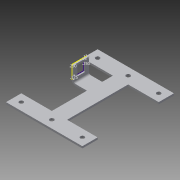
# Autodesk Inventor part: Cylinder Mount 2
Saved by Autodesk Inventor 2013 (Build 170138000, 138)
## iProperties
Created: 2013-01-26
Part Number: Cylinder Mount 2
Material: Aluminum 6061
Document SubType Name: Sheet Metal
Designer: actoennies
Density: 2.71 g/cm^3
Sheet Metal Rule: Default
Mass: 86.379 g
Surface Area: 232.571 cm^2
Volume: 31.8742 cm^3
Flat Pattern Width: 12.7 cm
Flat Pattern Length: 15.24 cm
Flat Pattern Area: 193.548 cm^2
Sheet Metal Width: 5.000 in
Sheet Metal Length: 6.000 in
Sheet Metal Area: 30.000 in^2
Author: actoennies
Autodesk Inventor part; units mm, degrees
ref_plane "YZ Plane" through (0, 0, 0) normal (1, 0, 0) x (0, 1, 0)
ref_plane "XZ Plane" through (0, 0, 0) normal (0, 1, 0) x (-1, 0, 0)
ref_plane "XY Plane" through (0, 0, 0) normal (0, 0, 1) x (1, 0, 0)
sketch "Sketch1" plane through (0, 0, 0) normal (1, 0, 0) x (0, 1, 0)
  line L0 (0, 0) -> (25.4, 0)
  line L1 (25.4, 0) -> (25.4, 25.4)
  line L2 (25.4, 25.4) -> (0, 25.4)
  line L3 (0, 25.4) -> (0, 0)
  dimension "d0" = 25.4
  dimension "d2" = 25.4
  measures "d0" distance of L1.end L2.end
  measures "d2" distance of L0.end L1.end
extrude "Plate1" add sketch "Sketch1" along normal blind 3.175
sketch "Sketch2" plane through (3.175, 0, 0) normal (0, -1, 0) x (1, 0, 0)
  line L0 (0, 25.4) -> (0, 0)
  line L1 (0, 0) -> (22.225, 0)
  line L2 (22.225, 0) -> (22.225, 25.4)
  line L3 (22.225, 25.4) -> (0, 25.4)
  constraints: 6 end point, 1 horizontal, 1 perpendicular, 1 vertical
edge flange "Flange1" height 25.4 angle 90 thickness 3.175 bend radius 3.175 thickness toward (0, -1, 0) relief straight relief width 3.175 relief depth 1.5875 edges at (3.175, 0, 12.7) wall of the first edge with corners at (3.175, 0, 25.4) (3.175, 0, 0) (25.4, 0, 0) (25.4, 0, 25.4)
bend "Bend1"
corner "Corner1"
sketch "Sketch3" plane through (25.4, 0, 25.4) normal (0, 1, 0) x (1, 0, 0)
  line L0 (0, 0) -> (0, 25.4)
  line L1 (0, 25.4) -> (-19.05, 25.4)
  line L2 (0, 0) -> (0, -83.82)
  line L3 (0, -83.82) -> (25.4, -83.82)
  line L4 (25.4, -83.82) -> (25.4, 68.58)
  line L5 (25.4, 68.58) -> (0, 68.58)
  line L6 (0, 68.58) -> (0, 25.4)
  point P0 (-25.4, 25.4)
  dimension "d14" = 83.82
  dimension "d15" = 25.4
  dimension "d16" = 152.4
  measures "d14" distance of L0.start L2.end
  measures "d15" distance of L2.end L3.end
  measures "d16" distance of L3.end L4.end
sheet face with bend "Face2" sketch "Sketch3" thickness 3.175 toward (0, -1, 0) bend radius 3.175 relief straight relief width 3.175 relief depth 1.5875
bend "Bend2"
sketch "Sketch4" plane through (0, 0, 0) normal (-1, 0, 0) x (0, 0, 1)
  line L0 (25.4, 25.4) -> (25.4, 3.175) projected
  line L1 (0, 25.4) -> (25.4, 25.4) projected
  line L2 (0, 3.175) -> (25.4, 3.175) projected
  line L3 (0, 3.175) -> (0, 25.4) projected
  line L4 (19.05, 22.225) -> (19.05, 6.35)
  line L5 (6.35, 22.225) -> (6.35, 6.35)
  line L6 (6.35, 6.35) -> (19.05, 6.35)
  line L7 (6.35, 22.225) -> (19.05, 22.225)
  point P0 (0, 0)
  dimension "d63" = 6.35
  dimension "d64" = 6.35
  dimension "d65" = 3.175
  dimension "d66" = 3.175
  constraints: 8 end point, 3 parallel, 1 perpendicular
  measures "d63" distance between parallel lines of L3 L5
  measures "d64" distance between parallel lines of L0 L4
  measures "d65" distance between parallel lines of L2 L6
  measures "d66" distance between parallel lines of L1 L7
sketch "Sketch5" plane through (6.35, 0, 25.4) normal (0, 1, 0) x (1, 0, 0)
  line L0 (19.05, -83.82) -> (44.45, -83.82) projected
  line L1 (44.45, -83.82) -> (44.45, 68.58) projected
  line L2 (44.45, 68.58) -> (19.05, 68.58) projected
  circle A0 centre (31.75, -71.12) radius 3.3782
  circle A1 centre (31.75, 55.88) radius 3.3782
  point P0 (-6.35, 25.4)
  dimension "d27" = 6.7564
  dimension "d28" = 12.7
  dimension "d29" = 12.7
  dimension "d30" = 6.7564
  dimension "d31" = 12.7
  dimension "d32" = 12.7
  constraints: 2 centre point
  measures "d27" diameter of A0
  measures "d28" distance from line of L1 A0.centre
  measures "d29" distance from line of L0 A0.centre
  measures "d30" diameter of A1
  measures "d31" distance from line of L2 A1.centre
  measures "d32" distance from line of L1 A1.centre
extrude "Cut2" cut sketch "Sketch5" against normal blind 3.175
sketch "Sketch6" plane through (6.35, -3.175, 0) normal (0, -1, 0) x (1, 0, 0)
  line L0 (19.05, -43.18) -> (19.05, 0)
  line L1 (44.45, -43.18) -> (19.05, -43.18)
  line L2 (44.45, 109.22) -> (44.45, -43.18)
  line L3 (19.05, 25.4) -> (19.05, 109.22)
  line L4 (0, 25.4) -> (19.05, 25.4)
  line L5 (19.05, -17.78) -> (-31.75, -17.78)
  line L6 (-31.75, -17.78) -> (-31.75, -43.18)
  line L7 (-31.75, -43.18) -> (19.05, -43.18)
  line L8 (19.05, 109.22) -> (-31.75, 109.22)
  line L9 (-31.75, 109.22) -> (-31.75, 83.82)
  line L10 (-31.75, 83.82) -> (19.05, 83.82)
  line L11 (44.45, 109.22) -> (95.25, 109.22)
  line L12 (95.25, 109.22) -> (95.25, 83.82)
  line L13 (95.25, 83.82) -> (44.45, 83.82)
  line L14 (44.45, -17.78) -> (95.25, -17.78)
  line L15 (95.25, -17.78) -> (95.25, -43.18)
  line L16 (95.25, -43.18) -> (44.45, -43.18)
  circle A0 centre (-19.05, 96.52) radius 3.3782
  circle A1 centre (82.55, 96.52) radius 3.3782
  circle A2 centre (-19.05, -30.48) radius 3.3782
  circle A3 centre (82.55, -30.48) radius 3.3782
  point P0 (-6.35, 0)
  dimension "d35" = 50.8
  dimension "d36" = 25.4
  dimension "d37" = 25.4
  dimension "d38" = 50.8
  dimension "d39" = 25.4
  dimension "d40" = 50.8
  dimension "d41" = 50.8
  dimension "d42" = 25.4
  dimension "d43" = 50.8
  dimension "d44" = 50.8
  dimension "d45" = 25.4
  dimension "d46" = 6.7564
  dimension "d47" = 6.7564
  dimension "d48" = 6.7564
  dimension "d49" = 6.7564
  dimension "d50" = 12.7
  dimension "d51" = 12.7
  dimension "d52" = 12.7
  dimension "d53" = 12.7
  dimension "d54" = 12.7
  dimension "d55" = 12.7
  dimension "d56" = 12.7
  dimension "d57" = 12.7
  measures "d35" distance of L5.start L5.end
  measures "d36" distance of L5.end L6.end
  measures "d37" distance from line of L1 L5.start
  measures "d38" distance of L3.end L8.end
  measures "d39" distance of L8.end L9.end
  measures "d40" distance of L9.end L10.end
  measures "d41" distance of L2.start L11.end
  measures "d42" distance of L11.end L12.end
  measures "d43" distance of L12.end L13.end
  measures "d44" distance of L14.start L14.end
  measures "d45" distance of L14.end L15.end
  measures "d46" diameter of A0
  measures "d47" diameter of A1
  measures "d48" diameter of A2
  measures "d49" diameter of A3
  measures "d50" distance from line of L6 A2.centre
  measures "d51" distance from line of L7 A2.centre
  measures "d52" distance from line of L15 A3.centre
  measures "d53" distance from line of L16 A3.centre
  measures "d54" distance from line of L11 A1.centre
  measures "d55" distance from line of L12 A1.centre
  measures "d56" distance from line of L8 A0.centre
  measures "d57" distance from line of A0.centre L9
sheet face with bend "Face3" sketch "Sketch6" thickness 3.175 toward (0, 1, 0) bend radius 3.175 relief straight relief width 3.175 relief depth 1.5875
bend "Bend3"
extrude "Cut3" cut sketch "Sketch4" against normal blind 3.175 contours L4 L6 L5 L7
equation "\"d33\" = Thickness"
equation "\"d67\" = Thickness"
equation "\"d4\" = BendReliefWidth"
equation "\"d5\" = BendReliefDepth"
equation "\"d6\" = MinimumRemnant"
equation "\"d7\" = BendRadius"
equation "\"d10\" = BendRadius"
equation "\"d11\" = CornerReliefSize"
equation "\"d12\" = GapSize"
equation "\"d13\" = JacobiRadiusSize"
equation "\"d17\" = BendRadius"
equation "\"d18\" = BendReliefWidth"
equation "\"d20\" = MinimumRemnant"
equation "\"d19\" = BendReliefDepth"
equation "\"d21\" = BendRadius"
equation "\"d58\" = BendRadius"
equation "\"d59\" = BendReliefWidth"
equation "\"d61\" = MinimumRemnant"
equation "\"d60\" = BendReliefDepth"
equation "\"d62\" = BendRadius"
equation "\"BendRadius\" = Thickness"
equation "\"BendReliefWidth\" = Thickness"
equation "\"BendReliefDepth\" = 0.5 * Thickness"
equation "\"CornerReliefSize\" = 4 * Thickness"
equation "\"MinimumRemnant\" = 2 * Thickness"
equation "\"TransitionRadius\" = BendRadius"
equation "\"JacobiRadiusSize\" = BendRadius"
equation "\"GapSize\" = Thickness"
equation "\"d3\" = BendRadius"
equation "\"Thickness\" = 3.175"
body "Solid1"
